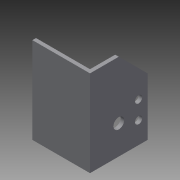
# Autodesk Inventor part: mechanical stop 2x2 angle
Saved by Autodesk Inventor 2015 SP1 (Build 190203100, 203)
## iProperties
Created: 2015-01-28
Part Number: mechanical stop 2x2 angle
Material: Generic
Document SubType Name: Modeling
Designer: Admin
Density: 1 g/cm^3
Appearance: Default
Author: Admin
Autodesk Inventor part; units mm, degrees
ref_plane "YZ Plane" through (0, 0, 0) normal (1, 0, 0) x (0, 1, 0)
ref_plane "XZ Plane" through (0, 0, 0) normal (0, 1, 0) x (-1, 0, 0)
ref_plane "XY Plane" through (0, 0, 0) normal (0, 0, 1) x (1, 0, 0)
sketch "Sketch1" plane through (0, 0, 0) normal (0, 1, 0) x (-1, 0, 0)
  line L0 (0, 0) -> (50.8, 0)
  line L1 (50.8, 0) -> (50.8, -3.175)
  line L2 (50.8, -3.175) -> (0, -3.175)
  line L3 (0, -3.175) -> (0, 0)
  line L4 (0, 0) -> (3.175, 0)
  line L5 (3.175, 0) -> (3.175, -50.8)
  line L6 (3.175, -50.8) -> (0, -50.8)
  line L7 (0, -50.8) -> (0, 0)
  dimension "d0" = 50.8
  dimension "d1" = 3.175
  dimension "d2" = 3.175
  dimension "d3" = 50.8
  constraints: 16 end point, 4 parallel, 2 horizontal, 2 perpendicular
  measures "d0" distance of L1.end L2.end
  measures "d1" distance of L0.end L1.end
  measures "d2" distance of L5.end L6.end
  measures "d3" distance of L4.end L5.end
extrude "Extrusion1" add sketch "Sketch1" along normal blind 76.2
sketch "Sketch4" plane through (0, 0, 0) normal (1, 0, 0) x (0, 0, -1)
  line L0 (0, 0) -> (0, 76.2) projected
  line L1 (0, 0) -> (50.8, 0) projected
  point P0 (25.4, 25.4)
  dimension "d11" = 25.4
  dimension "d12" = 25.4
  measures "d11" distance from line of L1 point (25.4, 25.4)
  measures "d12" distance from line of point (25.4, 25.4) L0
hole "Hole1" at (0, 25.4, -25.4) direction (-1, 0, 0) diameter 9.525 end through all
sketch "Sketch5" plane through (-3.175, 0, -50.8) normal (-1, 0, 0) x (0, 0, 1)
  circle A0 centre (25.4, 25.4) radius 4.7625 projected
  line L0 (0, 0) -> (0, 76.2) projected
  point P0 (50.8, 0)
  point P1 (7.9375, 19.05)
  point P2 (7.9375, 34.925)
  dimension "d20" = 9.525
  dimension "d21" = 6.35
  dimension "d23" = 7.9375
  dimension "d24" = 7.9375
  measures "d20" vertical distance of A0.centre point (7.938, 34.925)
  measures "d21" vertical distance of A0.centre point (7.938, 19.05)
  measures "d23" distance from line of L0 point (7.938, 19.05)
  measures "d24" distance from line of L0 point (7.938, 34.925)
hole "Hole2" at (-3.175, 19.05, -42.8625) at (-3.175, 34.925, -42.8625) direction (1, 0, 0) diameter 6.35 end through all
sketch "Sketch6" plane through (0, 0, 0) normal (1, 0, 0) x (0, 0, -1)
  line L0 (50.8, 0) -> (50.8, 76.2) projected
  line L1 (50.8, 76.2) -> (25.4, 76.2) construction
  line L2 (50.8, 76.2) -> (3.175, 76.2) construction
  line L3 (25.4, 76.2) -> (50.8, 50.8)
  line L4 (25.4, 76.2) -> (61.321, 76.2) construction
  line L5 (50.8, 50.8) -> (50.8, 76.2)
  line L6 (50.8, 76.2) -> (25.4, 76.2)
  dimension "d32" = 25.4
  dimension "d33" = 45
  constraints: 10 end point, 2 point on line, 1 collinear, 1 equal length, 1 horizontal, 1 vertical
  measures "d32" distance of L0.end L1.end
  measures "d33" angle of L3 L4
extrude "Extrusion4" cut sketch "Sketch6" against normal blind 76.2
body "Solid1"
